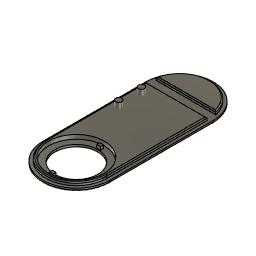
Krabicka pro termostat - víčko (Autodesk Fusion 360 design; units mm, degrees)
Autodesk Fusion 360 part; units mm, degrees
sketch "Sketch1" plane through (0, 0, 0) normal (0, 0, 1) x (1, 0, 0)
  circle A0 centre (0.0005, 0) radius 20.75
  arc A1 (32.4989, 100) -> (-32.5011, 100) centre (-0.0011, 100) ccw
  circle A2 centre (0.0005, 0) radius 27
  line L0 (-49, 0) -> (63, 0) construction
  line L1 (-32.5011, 100) -> (-32.4995, 0)
  line L2 (32.4989, 100) -> (32.5005, 0)
  arc A3 (-32.4995, 0) -> (32.5005, 0.0005) centre (0.0005, 0) ccw
  arc A4 (-29.5001, 0) -> (29.5005, 0) centre (0.0002, 0) ccw
  line L3 (-29.4995, 61.5) -> (-29.4995, 87.5)
  line L4 (-29.5011, 97) -> (29.4989, 97)
  line L5 (-28.8845, 106) -> (28.8823, 106)
  arc A5 (28.8823, 106) -> (-28.8845, 106) centre (-0.0011, 100) ccw
  line L6 (29.4989, 100.0007) -> (29.4989, 100)
  line L7 (29.4989, 97) -> (29.5005, 0)
  line L8 (-29.5011, 97) -> (-29.5001, 0)
  line L9 (-24.4995, 23.2909) -> (-38.4097, 23.2907) construction
  line L10 (-29.5011, 97) -> (-29.5001, 0)
  line L11 (-26.4995, 112) -> (22.6043, 112) construction
  line L12 (0.0002, 0) -> (0.0007, -38) construction
  line L13 (-1.7495, 21.5) -> (-1.7496, 24.5)
  line L14 (1.7505, 21.5) -> (1.7504, 24.5)
  line L15 (1.7505, 21.5) -> (-1.7495, 21.5)
  line L16 (1.7504, 24.5) -> (-1.7496, 24.5)
  circle A6 centre (17.4994, 112.0003) radius 2.5
  circle A7 centre (-17.5011, 112) radius 2.5
  circle A8 centre (24.4992, 23.2913) radius 2.5
  circle A9 centre (-24.4995, 23.2909) radius 2.5
  line L17 (1.7504, -24.5) -> (-1.7496, -24.5)
  line L18 (-1.7495, -21.5) -> (-1.7496, -24.5)
  line L19 (1.7505, -21.5) -> (-1.7495, -21.5)
  line L20 (1.7505, -21.5) -> (1.7504, -24.5)
  line L21 (-24.9995, 61) -> (3.0005, 61) construction
  line L22 (3.0005, 61) -> (3.0005, 88) construction
  line L23 (3.0005, 88) -> (-24.9995, 88) construction
  line L24 (-24.9995, 88) -> (-24.9995, 61) construction
  circle A10 centre (-22.4995, 63.5) radius 3
  line L25 (-24.9995, 74.5) -> (3.0005, 74.5) construction
  circle A11 centre (-22.4995, 85.5) radius 3
  circle A12 centre (-0.0011, 92.75) radius 2.5
  dimension "d2" = 41.5
  dimension "d3" = 65
  dimension "d76" = 54
  dimension "d88" = 65
  dimension "d91" = 100
  dimension "d107" = 3
  dimension "d118" = 26
  dimension "d144" = 5
  dimension "d145" = 8
  dimension "d148" = 5
  dimension "d149" = 4.25
  dimension "d150" = 32.5
  dimension "d151" = 5
  dimension "d152" = 15
  dimension "d153" = 12
  dimension "d235" = 21.5
  dimension "d236" = 3
  dimension "d237" = 27
  dimension "d238" = 28
  dimension "d239" = 6
  dimension "d243" = 2.5
  dimension "d244" = 2.5
  dimension "d245" = 61
  dimension "d246" = 25
  constraint concentric A0 A2
  constraint horizontal L0
  constraint concentric A0 A3
  constraint coincident L0 L1.end
  constraint coincident L2.end A3
  constraint coincident L0 L2.end
  constraint coincident L2 A3.end
  constraint coincident L0 A4.start
  constraint parallel L2 L6
  constraint coincident L4.end L6
  constraint collinear L6 L7
  constraint coincident L9.start A9.centre
  constraint coincident A4.centre L12.start
  constraint parallel L15 L16
  constraint symmetric L0 L13.start L18.start
  constraint symmetric L0 L13.end L17.end
  constraint symmetric L0 L14.start L19.start
  constraint symmetric L0 L14.end L17.start
  constraint horizontal L21
  constraint vertical L22
  constraint horizontal L23
  constraint vertical L24
  constraint midpoint L24 L25.start
  constraint midpoint L22 L25.end
  constraint symmetric A10 L25 A11
  measures "d2" diameter of A0
  measures "d3" diameter of A1
  measures "d76" diameter of A2
  measures "d88" diameter of A3
  measures "d91" vertical distance of A1.centre A0.centre
  measures "d107" horizontal distance of L1.end L3.start
  measures "d118" distance of L3.end L3.start
  measures "d144" diameter of A9
  measures "d145" horizontal distance of L1.end L9.start
  measures "d148" diameter of A12
  measures "d149" vertical distance of L4.start A12.centre
  measures "d150" horizontal distance of A1.end A12.centre
  measures "d151" diameter of A7
  measures "d152" horizontal distance of A1.end A7.centre
  measures "d153" vertical distance of A1.end A7.centre
  measures "d235" vertical distance of A0.centre L14.start
  measures "d236" distance of L14.start L14.end
  measures "d237" distance of L21.start L23.end
  measures "d238" distance of L21.start L21.end
  measures "d239" diameter of A10
  measures "d243" horizontal distance of L23.end A10.centre
  measures "d244" vertical distance of L21.start A10.centre
  measures "d245" vertical distance of A0.centre L21.start
  measures "d246" horizontal distance of A0.centre L21.start
extrude "Extrude30" add sketch "Sketch1" along normal blind 3 contours A1 L1 L2 A3 makes body 1
extrude "Extrude32" add sketch "Sketch1" along normal blind 5 separate body contours L13 L14 L15 L16 | L17 L18 L19 L20 makes body 2 at (-0.5829, 21.5, 3.3333) makes body 3 at (0.5838, -21.5, 1.6667)
extrude "Extrude33" add sketch "Sketch1" along normal blind 2 separate body contours A2 makes body 4
extrude "Extrude34" add sketch "Sketch1" along normal blind 6 separate body contours A4 L3 L4 L7 L8 L10 | L5 A5 | A6 | A7 | A8 | A9 | A10 | A11 | A12 makes body 5 at (-1.0934, 115.1669, 0) makes body 6 at (-0.6731, 73.6415, 0)
chamfer "Chamfer1" distance 1 angle 45 4 edges at (-29.5006, 48.5, 6) (0.0002, -29.5003, 6) (29.4997, 48.5, 6) (-0.0011, 97, 6) on bodies 6
chamfer "Chamfer2" distance 1 angle 45 2 edges at (-0.0011, 129.5, 6) (-0.0011, 106, 6) on bodies 5
fillet "Fillet1" radius 1.5 4 edges at (0.0007, -32.5, 0) (-32.5003, 50, 0) (-0.0011, 132.5, 0) (32.4997, 50.0003, 0) on bodies 1
extrude "Extrude35" cut sketch "Sketch1" along normal blind 2 contours A6 | A7 bodies 5
extrude "Extrude36" cut sketch "Sketch1" along normal blind 2 contours A8 | A9 bodies 6
extrude "Extrude37" cut sketch "Sketch1" along normal blind 2 contours A12 bodies 6
extrude "Extrude38" add sketch "Sketch1" along normal blind 11 separate body contours A10 | A11 makes body 7 at (-19.8649, 64.9348, 3.6667) makes body 8 at (-19.6805, 84.4739, 7.3333)
extrude "Extrude6" [suppressed]
extrude "Extrude7" [suppressed]
sketch "Sketch3" plane through (-30, 0, 0) normal (-1, 0, 0) x (0, -1, 0)
  line L0 (-60, 0) -> (0, 0)
  line L1 (0, 0) -> (0, 36)
  line L2 (0, 36) -> (-60, 36)
  line L3 (-60, 36) -> (-60, 0)
  line L4 (-52, 8) -> (-52, 28)
  line L5 (-55, 28) -> (-55, 8)
  arc A0 (-52, 28) -> (-55, 28) centre (-53.5, 28) ccw
  arc A1 (-55, 8) -> (-52, 8) centre (-53.5, 8) ccw
  arc A2 (-46.125, 28) -> (-49.125, 28) centre (-47.625, 28) ccw
  line L6 (-46.125, 8) -> (-46.125, 28)
  line L7 (-49.125, 28) -> (-49.125, 8)
  arc A3 (-49.125, 8) -> (-46.125, 8) centre (-47.625, 8) ccw
  arc A4 (-40.25, 28) -> (-43.25, 28) centre (-41.75, 28) ccw
  line L8 (-40.25, 8) -> (-40.25, 28)
  line L9 (-43.25, 28) -> (-43.25, 8)
  arc A5 (-43.25, 8) -> (-40.25, 8) centre (-41.75, 8) ccw
  arc A6 (-34.375, 28) -> (-37.375, 28) centre (-35.875, 28) ccw
  line L10 (-34.375, 8) -> (-34.375, 28)
  line L11 (-37.375, 28) -> (-37.375, 8)
  arc A7 (-37.375, 8) -> (-34.375, 8) centre (-35.875, 8) ccw
  arc A8 (-28.5, 28) -> (-31.5, 28) centre (-30, 28) ccw
  line L12 (-28.5, 8) -> (-28.5, 28)
  line L13 (-31.5, 28) -> (-31.5, 8)
  arc A9 (-31.5, 8) -> (-28.5, 8) centre (-30, 8) ccw
  arc A10 (-22.625, 28) -> (-25.625, 28) centre (-24.125, 28) ccw
  line L14 (-22.625, 8) -> (-22.625, 28)
  line L15 (-25.625, 28) -> (-25.625, 8)
  arc A11 (-25.625, 8) -> (-22.625, 8) centre (-24.125, 8) ccw
  arc A12 (-16.75, 28) -> (-19.75, 28) centre (-18.25, 28) ccw
  line L16 (-16.75, 8) -> (-16.75, 28)
  line L17 (-19.75, 28) -> (-19.75, 8)
  arc A13 (-19.75, 8) -> (-16.75, 8) centre (-18.25, 8) ccw
  arc A14 (-10.875, 28) -> (-13.875, 28) centre (-12.375, 28) ccw
  line L18 (-10.875, 8) -> (-10.875, 28)
  line L19 (-13.875, 28) -> (-13.875, 8)
  arc A15 (-13.875, 8) -> (-10.875, 8) centre (-12.375, 8) ccw
  arc A16 (-5, 28) -> (-8, 28) centre (-6.5, 28) ccw
  line L20 (-5, 8) -> (-5, 28)
  line L21 (-8, 28) -> (-8, 8)
  arc A17 (-8, 8) -> (-5, 8) centre (-6.5, 8) ccw
  line L22 (-60, 18) -> (-55, 18)
  dimension "d42" = 3
  dimension "d43" = 20
  dimension "d44" = 3
  dimension "d45" = 3
  dimension "d46" = 10
  dimension "d47" = 5
  dimension "d50" = 47
  dimension "d51" = 0
  constraint vertical L4
  constraint vertical L5
  constraint midpoint L3 L22.start
  constraint coincident L5 L22.end
  measures "d42" distance of L5.end L4.start
  measures "d43" distance of L5.end L5.start
  measures "d44" diameter of A1
  measures "d45" diameter of A0
  measures "d46" vertical distance of A0.centre L22.start
  measures "d47" horizontal distance of L5.end L22.start
extrude "Extrude8" [suppressed]
extrude "Extrude9" [suppressed]
